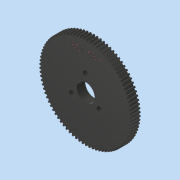
# Autodesk Inventor part: pistonSpurGear
Saved by Autodesk Inventor 2017 (Build 210142000, 142)
## iProperties
Created: 2016-11-28
Part Number: pistonSpurGear
Material: ABS Plastic
Document SubType Name: Modeling
Designer: techn
Density: 1.06 g/cm^3
Appearance: Smooth - Black
Author: techn
Autodesk Inventor part; units mm, degrees
ref_plane "YZ Plane" through (0, 0, 0) normal (1, 0, 0) x (0, 1, 0)
ref_plane "XZ Plane" through (0, 0, 0) normal (0, 1, 0) x (-1, 0, 0)
ref_plane "XY Plane" through (0, 0, 0) normal (0, 0, 1) x (1, 0, 0)
sketch "Sketch1" plane through (0, 0, 0) normal (0, 0, 1) x (1, 0, 0)
  circle A0 centre (0, 0) radius 23.114
  dimension "d0" = 46.228
  constraints: 1 centre point, 1 coincident
  measures "d0" diameter of A0
extrude "Extrusion1" add sketch "Sketch1" along normal blind 4.445
sketch "Sketch2" plane through (0, 0, 0) normal (0, 0, -1) x (-1, 0, 0)
  line L0 (0, 0) -> (0, 8.3295)
  circle A0 centre (0, 8.3295) radius 1.5875
  circle A1 centre (-7.2136, -4.1648) radius 1.5875
  circle A2 centre (7.2136, -4.1648) radius 1.5875
  dimension "d3" = 3.175
  dimension "d6" = 360
  dimension "d8" = 14.4272
  constraints: 3 centre point, 2 end point, 1 coincident, 1 vertical, 7 other
  measures "d3" diameter of A0
  measures "d8" distance of A2.centre L0.end
extrude "Extrusion2" cut sketch "Sketch2" against normal through all
sketch "Sketch3" plane through (0, 0, 4.445) normal (0, 0, 1) x (1, 0, 0)
  circle A0 centre (0, 0) radius 4.7625
  dimension "d11" = 9.525
  constraints: 1 centre point, 1 coincident
  measures "d11" diameter of A0
extrude "Extrusion3" cut sketch "Sketch3" against normal through all
sketch "Sketch4" plane through (0, 0, 4.445) normal (0, 0, 1) x (1, 0, 0)
  line L0 (-0.2667, 24.0763) -> (0.2667, 24.0763)
  line L1 (0.2667, 24.0763) -> (0.3683, 23.4921)
  line L2 (0.3683, 23.4921) -> (0.3683, 23.1111)
  line L3 (0.3683, 23.1111) -> (-0.3683, 23.1111)
  line L4 (-0.3683, 23.1111) -> (-0.3683, 23.4921)
  line L5 (-0.3683, 23.4921) -> (-0.2667, 24.0763)
  circle A0 centre (0, 0) radius 23.114 construction
  point P0 (0, 24.0763)
  dimension "d14" = 0.5334
  dimension "d15" = 0.7366
  dimension "d16" = 0.9652
  dimension "d17" = 0.381
  constraints: 12 end point, 2 equal length, 2 perpendicular, 1 horizontal, 1 midpoint, 1 vertical, 1 vertical alignment, 2 other
  measures "d14" distance of L0.start L0.end
  measures "d15" distance of L2.end L3.end
  measures "d16" distance between parallel lines of L0 L3
  measures "d17" distance of L3.end L4.end
extrude "Extrusion4" add sketch "Sketch4" against normal up to surface (4.445 mm away)
pattern_circular "Circular Pattern1" count 86 over 360 about axis through (0, 0, 0) along (0, 0, 1) of "Extrusion4"
sketch "Sketch5" plane through (0, 0, 4.445) normal (0, 0, 1) x (1, 0, 0)
  line L0 (-7.6264, 19.8299) -> (7.5914, 19.8299) construction
  line L1 (7.5914, 19.8299) -> (7.5914, 16.6436) construction
  line L2 (7.5914, 16.6436) -> (-7.6264, 16.6436) construction
  line L3 (-7.6264, 16.6436) -> (-7.6264, 19.8299) construction
  spline S0 degree 2 poles (-6.4828, 16.6436) (-6.71, 16.6436) (-7.083, 16.7794) (-7.2139, 16.9054) knots 0 0 0 1 2 2 2
  spline S1 degree 2 poles (-7.2139, 16.9054) (-7.3424, 17.0289) (-7.4757, 17.3648) (-7.4757, 17.555) knots 0 0 0 1 2 2 2
  spline S2 degree 2 poles (-7.4757, 17.555) (-7.4757, 17.802) (-7.2114, 18.217) (-6.9595, 18.3405) knots 0 0 0 1 2 2 2
  line L4 (-6.9595, 18.3405) -> (-6.9595, 18.3528)
  spline S3 degree 2 poles (-6.9595, 18.3528) (-7.1843, 18.4837) (-7.4016, 18.7949) (-7.4016, 19.0271) knots 0 0 0 1 2 2 2
  spline S4 degree 2 poles (-7.4016, 19.0271) (-7.4016, 19.3705) (-6.8829, 19.8299) (-6.4828, 19.8299) knots 0 0 0 1 2 2 2
  spline S5 degree 2 poles (-6.4828, 19.8299) (-6.0678, 19.8299) (-5.5664, 19.3952) (-5.5664, 19.0543) knots 0 0 0 1 2 2 2
  spline S6 degree 2 poles (-5.5664, 19.0543) (-5.5664, 18.8493) (-5.806, 18.4491) (-6.0308, 18.3355) knots 0 0 0 1 2 2 2
  line L5 (-6.0308, 18.3355) -> (-6.0308, 18.3232)
  spline S7 degree 2 poles (-6.0308, 18.3232) (-5.764, 18.1997) (-5.4898, 17.844) (-5.4898, 17.5624) knots 0 0 0 1 2 2 2
  spline S8 degree 2 poles (-5.4898, 17.5624) (-5.4898, 17.1721) (-6.0579, 16.6436) (-6.4828, 16.6436) knots 0 0 0 1 2 2 2
  spline S9 degree 2 poles (-5.9097, 17.5229) (-5.9097, 17.7106) (-6.0579, 17.9329) (-6.2679, 18.0465) knots 0 0 0 1 2 2 2
  spline S10 degree 2 poles (-6.2679, 18.0465) (-6.3371, 18.086) (-6.5692, 18.1774) (-6.715, 18.2367) knots 0 0 0 1 2 2 2
  spline S11 degree 2 poles (-6.715, 18.2367) (-6.8829, 18.1256) (-7.0632, 17.7946) (-7.0632, 17.5846) knots 0 0 0 1 2 2 2
  spline S12 degree 2 poles (-7.0632, 17.5846) (-7.0632, 17.308) (-6.7298, 16.9474) (-6.4778, 16.9474) knots 0 0 0 1 2 2 2
  spline S13 degree 2 poles (-6.4778, 16.9474) (-6.221, 16.9474) (-5.9097, 17.2561) (-5.9097, 17.5229) knots 0 0 0 1 2 2 2
  spline S14 degree 2 poles (-5.9666, 19.0493) (-5.9666, 19.2544) (-6.2407, 19.5285) (-6.4853, 19.5285) knots 0 0 0 1 2 2 2
  spline S15 degree 2 poles (-6.4853, 19.5285) (-6.7076, 19.5285) (-6.9916, 19.284) (-6.9916, 19.074) knots 0 0 0 1 2 2 2
  spline S16 degree 2 poles (-6.9916, 19.074) (-6.9916, 18.9234) (-6.8459, 18.7134) (-6.7001, 18.6294) knots 0 0 0 1 2 2 2
  spline S17 degree 2 poles (-6.7001, 18.6294) (-6.6384, 18.5949) (-6.3766, 18.4738) (-6.2704, 18.4393) knots 0 0 0 1 2 2 2
  spline S18 degree 2 poles (-6.2704, 18.4393) (-6.0925, 18.5751) (-5.9666, 18.8641) (-5.9666, 19.0493) knots 0 0 0 1 2 2 2
  spline S19 degree 2 poles (-3.1903, 17.7007) (-3.1903, 17.4661) (-3.3459, 17.0684) (-3.4768, 16.935) knots 0 0 0 1 2 2 2
  spline S20 degree 2 poles (-3.4768, 16.935) (-3.6126, 16.7942) (-3.9535, 16.6485) (-4.1585, 16.6485) knots 0 0 0 1 2 2 2
  spline S21 degree 2 poles (-4.1585, 16.6485) (-4.3635, 16.6485) (-4.7019, 16.7868) (-4.8303, 16.9251) knots 0 0 0 1 2 2 2
  spline S22 degree 2 poles (-4.8303, 16.9251) (-4.9884, 17.0906) (-5.1663, 17.6464) (-5.1663, 18.0515) knots 0 0 0 1 2 2 2
  spline S23 degree 2 poles (-5.1663, 18.0515) (-5.1663, 18.4491) (-5.0032, 19.0889) (-4.8328, 19.326) knots 0 0 0 1 2 2 2
  spline S24 degree 2 poles (-4.8328, 19.326) (-4.6673, 19.5582) (-4.1437, 19.8175) (-3.8003, 19.8175) knots 0 0 0 1 2 2 2
  spline S25 degree 2 poles (-3.8003, 19.8175) (-3.6991, 19.8175) (-3.5212, 19.7978) (-3.4545, 19.7755) knots 0 0 0 1 2 2 2
  line L6 (-3.4545, 19.7755) -> (-3.4545, 19.3828)
  line L7 (-3.4545, 19.3828) -> (-3.4718, 19.3828)
  spline S26 degree 2 poles (-3.4718, 19.3828) (-3.5286, 19.4124) (-3.7361, 19.4643) (-3.8547, 19.4643) knots 0 0 0 1 2 2 2
  spline S27 degree 2 poles (-3.8547, 19.4643) (-4.2351, 19.4643) (-4.7019, 18.9505) (-4.7464, 18.4467) knots 0 0 0 1 2 2 2
  spline S28 degree 2 poles (-4.7464, 18.4467) (-4.6006, 18.5479) (-4.2944, 18.6591) (-4.1116, 18.6591) knots 0 0 0 1 2 2 2
  spline S29 degree 2 poles (-4.1116, 18.6591) (-3.9337, 18.6591) (-3.667, 18.5875) (-3.5212, 18.4788) knots 0 0 0 1 2 2 2
  spline S30 degree 2 poles (-3.5212, 18.4788) (-3.3533, 18.3528) (-3.1903, 17.9625) (-3.1903, 17.7007) knots 0 0 0 1 2 2 2
  spline S31 degree 2 poles (-3.6052, 17.6834) (-3.6052, 17.8712) (-3.704, 18.1256) (-3.8127, 18.2145) knots 0 0 0 1 2 2 2
  spline S32 degree 2 poles (-3.8127, 18.2145) (-3.8942, 18.2787) (-4.0967, 18.3207) (-4.203, 18.3207) knots 0 0 0 1 2 2 2
  spline S33 degree 2 poles (-4.203, 18.3207) (-4.3462, 18.3207) (-4.6155, 18.2342) (-4.7464, 18.1527) knots 0 0 0 1 2 2 2
  spline S34 degree 2 poles (-4.7464, 18.1527) (-4.7488, 18.1083) (-4.7538, 18.0243) (-4.7538, 17.9601) knots 0 0 0 1 2 2 2
  spline S35 degree 2 poles (-4.7538, 17.9601) (-4.7538, 17.6439) (-4.6303, 17.2561) (-4.5364, 17.1548) knots 0 0 0 1 2 2 2
  spline S36 degree 2 poles (-4.5364, 17.1548) (-4.45, 17.0585) (-4.2622, 16.9819) (-4.156, 16.9819) knots 0 0 0 1 2 2 2
  spline S37 degree 2 poles (-4.156, 16.9819) (-3.909, 16.9819) (-3.6052, 17.3327) (-3.6052, 17.6834) knots 0 0 0 1 2 2 2
  line L8 (-2.0318, 16.7127) -> (-2.0318, 19.4001)
  line L9 (-2.0318, 19.4001) -> (-3.0544, 19.4001)
  line L10 (-3.0544, 19.4001) -> (-3.0544, 19.7607)
  line L11 (-3.0544, 19.7607) -> (-0.6041, 19.7607)
  line L12 (-0.6041, 19.7607) -> (-0.6041, 19.4001)
  line L13 (-0.6041, 19.4001) -> (-1.6267, 19.4001)
  line L14 (-1.6267, 19.4001) -> (-1.6267, 16.7127)
  line L15 (-1.6267, 16.7127) -> (-2.0318, 16.7127)
  line L16 (2.8885, 17.76) -> (2.5254, 17.76)
  line L17 (2.5254, 17.76) -> (2.5254, 16.7127)
  line L18 (2.5254, 16.7127) -> (2.1326, 16.7127)
  line L19 (2.1326, 16.7127) -> (2.1326, 17.76)
  line L20 (2.1326, 17.76) -> (0.7865, 17.76)
  line L21 (0.7865, 17.76) -> (0.7865, 18.1898)
  line L22 (0.7865, 18.1898) -> (2.1499, 19.7607)
  line L23 (2.1499, 19.7607) -> (2.5254, 19.7607)
  line L24 (2.5254, 19.7607) -> (2.5254, 18.0885)
  line L25 (2.5254, 18.0885) -> (2.8885, 18.0885)
  line L26 (2.8885, 18.0885) -> (2.8885, 17.76)
  line L27 (2.1326, 18.0885) -> (2.1326, 19.2791)
  line L28 (2.1326, 19.2791) -> (1.1076, 18.0885)
  line L29 (1.1076, 18.0885) -> (2.1326, 18.0885)
  spline S38 degree 2 poles (4.1358, 16.6436) (3.9086, 16.6436) (3.5356, 16.7794) (3.4047, 16.9054) knots 0 0 0 1 2 2 2
  spline S39 degree 2 poles (3.4047, 16.9054) (3.2762, 17.0289) (3.1429, 17.3648) (3.1429, 17.555) knots 0 0 0 1 2 2 2
  spline S40 degree 2 poles (3.1429, 17.555) (3.1429, 17.802) (3.4072, 18.217) (3.6591, 18.3405) knots 0 0 0 1 2 2 2
  line L30 (3.6591, 18.3405) -> (3.6591, 18.3528)
  spline S41 degree 2 poles (3.6591, 18.3528) (3.4343, 18.4837) (3.217, 18.7949) (3.217, 19.0271) knots 0 0 0 1 2 2 2
  spline S42 degree 2 poles (3.217, 19.0271) (3.217, 19.3705) (3.7357, 19.8299) (4.1358, 19.8299) knots 0 0 0 1 2 2 2
  spline S43 degree 2 poles (4.1358, 19.8299) (4.5508, 19.8299) (5.0522, 19.3952) (5.0522, 19.0543) knots 0 0 0 1 2 2 2
  spline S44 degree 2 poles (5.0522, 19.0543) (5.0522, 18.8493) (4.8126, 18.4491) (4.5878, 18.3355) knots 0 0 0 1 2 2 2
  line L31 (4.5878, 18.3355) -> (4.5878, 18.3232)
  spline S45 degree 2 poles (4.5878, 18.3232) (4.8546, 18.1997) (5.1288, 17.844) (5.1288, 17.5624) knots 0 0 0 1 2 2 2
  spline S46 degree 2 poles (5.1288, 17.5624) (5.1288, 17.1721) (4.5607, 16.6436) (4.1358, 16.6436) knots 0 0 0 1 2 2 2
  spline S47 degree 2 poles (4.7089, 17.5229) (4.7089, 17.7106) (4.5607, 17.9329) (4.3507, 18.0465) knots 0 0 0 1 2 2 2
  spline S48 degree 2 poles (4.3507, 18.0465) (4.2815, 18.086) (4.0494, 18.1774) (3.9036, 18.2367) knots 0 0 0 1 2 2 2
  spline S49 degree 2 poles (3.9036, 18.2367) (3.7357, 18.1256) (3.5554, 17.7946) (3.5554, 17.5846) knots 0 0 0 1 2 2 2
  spline S50 degree 2 poles (3.5554, 17.5846) (3.5554, 17.308) (3.8888, 16.9474) (4.1408, 16.9474) knots 0 0 0 1 2 2 2
  spline S51 degree 2 poles (4.1408, 16.9474) (4.3976, 16.9474) (4.7089, 17.2561) (4.7089, 17.5229) knots 0 0 0 1 2 2 2
  spline S52 degree 2 poles (4.652, 19.0493) (4.652, 19.2544) (4.3779, 19.5285) (4.1333, 19.5285) knots 0 0 0 1 2 2 2
  spline S53 degree 2 poles (4.1333, 19.5285) (3.911, 19.5285) (3.627, 19.284) (3.627, 19.074) knots 0 0 0 1 2 2 2
  spline S54 degree 2 poles (3.627, 19.074) (3.627, 18.9234) (3.7727, 18.7134) (3.9185, 18.6294) knots 0 0 0 1 2 2 2
  spline S55 degree 2 poles (3.9185, 18.6294) (3.9802, 18.5949) (4.242, 18.4738) (4.3482, 18.4393) knots 0 0 0 1 2 2 2
  spline S56 degree 2 poles (4.3482, 18.4393) (4.5261, 18.5751) (4.652, 18.8641) (4.652, 19.0493) knots 0 0 0 1 2 2 2
  spline S57 degree 2 poles (7.5148, 18.8419) (7.5148, 18.6443) (7.374, 18.2886) (7.248, 18.1651) knots 0 0 0 1 2 2 2
  spline S58 degree 2 poles (7.248, 18.1651) (7.09, 18.0095) (6.6626, 17.8489) (6.3366, 17.8489) knots 0 0 0 1 2 2 2
  line L32 (6.3366, 17.8489) -> (5.9933, 17.8489)
  line L33 (5.9933, 17.8489) -> (5.9933, 16.7127)
  line L34 (5.9933, 16.7127) -> (5.5882, 16.7127)
  line L35 (5.5882, 16.7127) -> (5.5882, 19.7607)
  line L36 (5.5882, 19.7607) -> (6.3539, 19.7607)
  spline S59 degree 2 poles (6.3539, 19.7607) (6.6256, 19.7607) (7.006, 19.6718) (7.1517, 19.5705) knots 0 0 0 1 2 2 2
  spline S60 degree 2 poles (7.1517, 19.5705) (7.3221, 19.4544) (7.5148, 19.0963) (7.5148, 18.8419) knots 0 0 0 1 2 2 2
  spline S61 degree 2 poles (7.0924, 18.8295) (7.0924, 18.9876) (6.9837, 19.2198) (6.8726, 19.2939) knots 0 0 0 1 2 2 2
  spline S62 degree 2 poles (6.8726, 19.2939) (6.7763, 19.3581) (6.5194, 19.41) (6.3292, 19.41) knots 0 0 0 1 2 2 2
  line L37 (6.3292, 19.41) -> (5.9933, 19.41)
  line L38 (5.9933, 19.41) -> (5.9933, 18.1947)
  line L39 (5.9933, 18.1947) -> (6.2699, 18.1947)
  spline S63 degree 2 poles (6.2699, 18.1947) (6.5169, 18.1947) (6.8207, 18.2738) (6.9195, 18.3775) knots 0 0 0 1 2 2 2
  spline S64 degree 2 poles (6.9195, 18.3775) (7.0109, 18.4689) (7.0924, 18.6838) (7.0924, 18.8295) knots 0 0 0 1 2 2 2
  point P0 (0, 0)
  constraints: 2 other
emboss "Emboss1" sketch "Sketch5" operation cut depth 0.254 direction (0, 0, -1)
body "Solid1"
